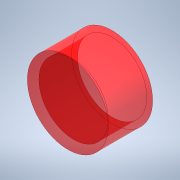
# Autodesk Inventor part: plastic diffuser
Saved by Autodesk Inventor 2022.1 (Build 261234000, 234)
## iProperties
Created: 2019-08-22
Part Number: plastic diffuser
Material: Стекло
Document SubType Name: Modeling
Designer: Иванов Д.А.
Mass: 3.13584 g
Surface Area: 20.169 cm^2
Volume: 1.43846 cm^3
Density: 2.18 g/cm^3
Appearance: Стеклянная лампа — Откл
Author: Иванов Д.А.
Autodesk Inventor part; units mm, degrees
(part 1 of 2)
ref_plane "YZ Plane" through (0, 0, 0) normal (1, 0, 0) x (0, 1, 0)
ref_plane "XZ Plane" through (0, 0, 0) normal (0, 1, 0) x (-1, 0, 0)
ref_plane "XY Plane" through (0, 0, 0) normal (0, 0, 1) x (1, 0, 0)
sketch "Эскиз1" plane through (0, 0, 0) normal (0, 1, 0) x (-1, 0, 0)
  circle A0 centre (0, 0) radius 9
  circle A1 centre (0, 0) radius 10.5
  dimension "d0" = 18
  dimension "d1" = 21
  constraints: 2 centre point, 2 coincident
  measures "d0" diameter of A0
  measures "d1" diameter of A1
extrude "Выдавливание1" add sketch "Эскиз1" along normal blind 10
extrude "Выдавливание2" add sketch "Эскиз1" against normal blind 1.5 contours A0 | A1
sketch "Эскиз3" plane through (0, 10, 0) normal (0, 1, 0) x (1, 0, 0)
  circle A0 centre (0, -9) radius 0.125
  circle A1 centre (0, 0) radius 9 projected
  line L0 (0, -9) -> (0, 0) construction
  line L1 (0, 0) -> (9, 0) construction
  circle A2 centre (0, -8.5) radius 0.125
  circle A3 centre (0, -8) radius 0.125
  circle A4 centre (0, -7.5) radius 0.125
  circle A5 centre (0, -7) radius 0.125
  circle A6 centre (0, -6.5) radius 0.125
  circle A7 centre (0, -6) radius 0.125
  circle A8 centre (0, -5.5) radius 0.125
  circle A9 centre (0, -5) radius 0.125
  circle A10 centre (0, -4.5) radius 0.125
  circle A11 centre (0, -4) radius 0.125
  circle A12 centre (0, -3.5) radius 0.125
  circle A13 centre (0, -3) radius 0.125
  circle A14 centre (0, -2.5) radius 0.125
  circle A15 centre (0, -2) radius 0.125
  circle A16 centre (0, -1.5) radius 0.125
  circle A17 centre (0, -1) radius 0.125
  circle A18 centre (0, -0.5) radius 0.125
  circle A19 centre (0, 0) radius 0.125
  circle A20 centre (0, 0.5) radius 0.125
  circle A21 centre (0, 1) radius 0.125
  circle A22 centre (0, 1.5) radius 0.125
  circle A23 centre (0, 2) radius 0.125
  circle A24 centre (0, 2.5) radius 0.125
  circle A25 centre (0, 3) radius 0.125
  circle A26 centre (0, 3.5) radius 0.125
  circle A27 centre (0, 4) radius 0.125
  circle A28 centre (0, 4.5) radius 0.125
  circle A29 centre (0, 5) radius 0.125
  circle A30 centre (0, 5.5) radius 0.125
  circle A31 centre (0, 6) radius 0.125
  circle A32 centre (0, 6.5) radius 0.125
  circle A33 centre (0, 7) radius 0.125
  circle A34 centre (0, 7.5) radius 0.125
  circle A35 centre (0, 8) radius 0.125
  circle A36 centre (0, 8.5) radius 0.125
  circle A37 centre (0, 9) radius 0.125
  circle A38 centre (0.5, -9) radius 0.125
  circle A39 centre (0.5, -8.5) radius 0.125
  circle A40 centre (0.5, -8) radius 0.125
  circle A41 centre (0.5, -7.5) radius 0.125
  circle A42 centre (0.5, -7) radius 0.125
  circle A43 centre (0.5, -6.5) radius 0.125
  circle A44 centre (0.5, -6) radius 0.125
  circle A45 centre (0.5, -5.5) radius 0.125
  circle A46 centre (0.5, -5) radius 0.125
  circle A47 centre (0.5, -4.5) radius 0.125
  circle A48 centre (0.5, -4) radius 0.125
  circle A49 centre (0.5, -3.5) radius 0.125
  circle A50 centre (0.5, -3) radius 0.125
  circle A51 centre (0.5, -2.5) radius 0.125
  circle A52 centre (0.5, -2) radius 0.125
  circle A53 centre (0.5, -1.5) radius 0.125
  circle A54 centre (0.5, -1) radius 0.125
  circle A55 centre (0.5, -0.5) radius 0.125
  circle A56 centre (0.5, 0) radius 0.125
  circle A57 centre (0.5, 0.5) radius 0.125
  circle A58 centre (0.5, 1) radius 0.125
  circle A59 centre (0.5, 1.5) radius 0.125
  circle A60 centre (0.5, 2) radius 0.125
  circle A61 centre (0.5, 2.5) radius 0.125
  circle A62 centre (0.5, 3) radius 0.125
  circle A63 centre (0.5, 3.5) radius 0.125
  circle A64 centre (0.5, 4) radius 0.125
  circle A65 centre (0.5, 4.5) radius 0.125
  circle A66 centre (0.5, 5) radius 0.125
  circle A67 centre (0.5, 5.5) radius 0.125
  circle A68 centre (0.5, 6) radius 0.125
  circle A69 centre (0.5, 6.5) radius 0.125
  circle A70 centre (0.5, 7) radius 0.125
  circle A71 centre (0.5, 7.5) radius 0.125
  circle A72 centre (0.5, 8) radius 0.125
  circle A73 centre (0.5, 8.5) radius 0.125
  circle A74 centre (0.5, 9) radius 0.125
  circle A75 centre (1, -9) radius 0.125
  circle A76 centre (1, -8.5) radius 0.125
  circle A77 centre (1, -8) radius 0.125
  circle A78 centre (1, -7.5) radius 0.125
  circle A79 centre (1, -7) radius 0.125
  circle A80 centre (1, -6.5) radius 0.125
  circle A81 centre (1, -6) radius 0.125
  circle A82 centre (1, -5.5) radius 0.125
  circle A83 centre (1, -5) radius 0.125
  circle A84 centre (1, -4.5) radius 0.125
  circle A85 centre (1, -4) radius 0.125
  circle A86 centre (1, -3.5) radius 0.125
  circle A87 centre (1, -3) radius 0.125
  circle A88 centre (1, -2.5) radius 0.125
  circle A89 centre (1, -2) radius 0.125
  circle A90 centre (1, -1.5) radius 0.125
  circle A91 centre (1, -1) radius 0.125
  circle A92 centre (1, -0.5) radius 0.125
  circle A93 centre (1, 0) radius 0.125
  circle A94 centre (1, 0.5) radius 0.125
  circle A95 centre (1, 1) radius 0.125
  circle A96 centre (1, 1.5) radius 0.125
  circle A97 centre (1, 2) radius 0.125
  circle A98 centre (1, 2.5) radius 0.125
  circle A99 centre (1, 3) radius 0.125
  circle A100 centre (1, 3.5) radius 0.125
  circle A101 centre (1, 4) radius 0.125
  circle A102 centre (1, 4.5) radius 0.125
  circle A103 centre (1, 5) radius 0.125
  circle A104 centre (1, 5.5) radius 0.125
  circle A105 centre (1, 6) radius 0.125
  circle A106 centre (1, 6.5) radius 0.125
  circle A107 centre (1, 7) radius 0.125
  circle A108 centre (1, 7.5) radius 0.125
  circle A109 centre (1, 8) radius 0.125
  circle A110 centre (1, 8.5) radius 0.125
  circle A111 centre (1, 9) radius 0.125
  circle A112 centre (1.5, -9) radius 0.125
  circle A113 centre (1.5, -8.5) radius 0.125
  circle A114 centre (1.5, -8) radius 0.125
  circle A115 centre (1.5, -7.5) radius 0.125
  circle A116 centre (1.5, -7) radius 0.125
  circle A117 centre (1.5, -6.5) radius 0.125
  circle A118 centre (1.5, -6) radius 0.125
  circle A119 centre (1.5, -5.5) radius 0.125
  circle A120 centre (1.5, -5) radius 0.125
  circle A121 centre (1.5, -4.5) radius 0.125
  circle A122 centre (1.5, -4) radius 0.125
  circle A123 centre (1.5, -3.5) radius 0.125
  circle A124 centre (1.5, -3) radius 0.125
  circle A125 centre (1.5, -2.5) radius 0.125
  circle A126 centre (1.5, -2) radius 0.125
  circle A127 centre (1.5, -1.5) radius 0.125
  circle A128 centre (1.5, -1) radius 0.125
  circle A129 centre (1.5, -0.5) radius 0.125
  circle A130 centre (1.5, 0) radius 0.125
  circle A131 centre (1.5, 0.5) radius 0.125
  circle A132 centre (1.5, 1) radius 0.125
  circle A133 centre (1.5, 1.5) radius 0.125
  circle A134 centre (1.5, 2) radius 0.125
  circle A135 centre (1.5, 2.5) radius 0.125
  circle A136 centre (1.5, 3) radius 0.125
  circle A137 centre (1.5, 3.5) radius 0.125
  circle A138 centre (1.5, 4) radius 0.125
  circle A139 centre (1.5, 4.5) radius 0.125
  circle A140 centre (1.5, 5) radius 0.125
  circle A141 centre (1.5, 5.5) radius 0.125
  circle A142 centre (1.5, 6) radius 0.125
  circle A143 centre (1.5, 6.5) radius 0.125
  circle A144 centre (1.5, 7) radius 0.125
  circle A145 centre (1.5, 7.5) radius 0.125
  circle A146 centre (1.5, 8) radius 0.125
  circle A147 centre (1.5, 8.5) radius 0.125
  circle A148 centre (1.5, 9) radius 0.125
  circle A149 centre (2, -9) radius 0.125
  circle A150 centre (2, -8.5) radius 0.125
  circle A151 centre (2, -8) radius 0.125
  circle A152 centre (2, -7.5) radius 0.125
  circle A153 centre (2, -7) radius 0.125
  circle A154 centre (2, -6.5) radius 0.125
  circle A155 centre (2, -6) radius 0.125
  circle A156 centre (2, -5.5) radius 0.125
  circle A157 centre (2, -5) radius 0.125
  circle A158 centre (2, -4.5) radius 0.125
  circle A159 centre (2, -4) radius 0.125
  circle A160 centre (2, -3.5) radius 0.125
  circle A161 centre (2, -3) radius 0.125
  circle A162 centre (2, -2.5) radius 0.125
  circle A163 centre (2, -2) radius 0.125
  circle A164 centre (2, -1.5) radius 0.125
  circle A165 centre (2, -1) radius 0.125
  circle A166 centre (2, -0.5) radius 0.125
  circle A167 centre (2, 0) radius 0.125
  circle A168 centre (2, 0.5) radius 0.125
  circle A169 centre (2, 1) radius 0.125
  circle A170 centre (2, 1.5) radius 0.125
  circle A171 centre (2, 2) radius 0.125
  circle A172 centre (2, 2.5) radius 0.125
  circle A173 centre (2, 3) radius 0.125
  circle A174 centre (2, 3.5) radius 0.125
  circle A175 centre (2, 4) radius 0.125
  circle A176 centre (2, 4.5) radius 0.125
  circle A177 centre (2, 5) radius 0.125
  circle A178 centre (2, 5.5) radius 0.125
  circle A179 centre (2, 6) radius 0.125
  circle A180 centre (2, 6.5) radius 0.125
  circle A181 centre (2, 7) radius 0.125
  circle A182 centre (2, 7.5) radius 0.125
  circle A183 centre (2, 8) radius 0.125
  circle A184 centre (2, 8.5) radius 0.125
  circle A185 centre (2, 9) radius 0.125
  circle A186 centre (2.5, -9) radius 0.125
  circle A187 centre (2.5, -8.5) radius 0.125
  circle A188 centre (2.5, -8) radius 0.125
  circle A189 centre (2.5, -7.5) radius 0.125
  circle A190 centre (2.5, -7) radius 0.125
  circle A191 centre (2.5, -6.5) radius 0.125
  circle A192 centre (2.5, -6) radius 0.125
  circle A193 centre (2.5, -5.5) radius 0.125
  circle A194 centre (2.5, -5) radius 0.125
  circle A195 centre (2.5, -4.5) radius 0.125
  circle A196 centre (2.5, -4) radius 0.125
  circle A197 centre (2.5, -3.5) radius 0.125
  circle A198 centre (2.5, -3) radius 0.125
  circle A199 centre (2.5, -2.5) radius 0.125
  circle A200 centre (2.5, -2) radius 0.125
  circle A201 centre (2.5, -1.5) radius 0.125
  circle A202 centre (2.5, -1) radius 0.125
  circle A203 centre (2.5, -0.5) radius 0.125
  circle A204 centre (2.5, 0) radius 0.125
  circle A205 centre (2.5, 0.5) radius 0.125
  circle A206 centre (2.5, 1) radius 0.125
  circle A207 centre (2.5, 1.5) radius 0.125
  circle A208 centre (2.5, 2) radius 0.125
  circle A209 centre (2.5, 2.5) radius 0.125
  circle A210 centre (2.5, 3) radius 0.125
  circle A211 centre (2.5, 3.5) radius 0.125
  circle A212 centre (2.5, 4) radius 0.125
  circle A213 centre (2.5, 4.5) radius 0.125
  circle A214 centre (2.5, 5) radius 0.125
  circle A215 centre (2.5, 5.5) radius 0.125
  circle A216 centre (2.5, 6) radius 0.125
  circle A217 centre (2.5, 6.5) radius 0.125
  circle A218 centre (2.5, 7) radius 0.125
  circle A219 centre (2.5, 7.5) radius 0.125
  circle A220 centre (2.5, 8) radius 0.125
  circle A221 centre (2.5, 8.5) radius 0.125
  circle A222 centre (2.5, 9) radius 0.125
  circle A223 centre (3, -9) radius 0.125
  circle A224 centre (3, -8.5) radius 0.125
  circle A225 centre (3, -8) radius 0.125
  circle A226 centre (3, -7.5) radius 0.125
  circle A227 centre (3, -7) radius 0.125
  circle A228 centre (3, -6.5) radius 0.125
  circle A229 centre (3, -6) radius 0.125
  circle A230 centre (3, -5.5) radius 0.125
  circle A231 centre (3, -5) radius 0.125
  circle A232 centre (3, -4.5) radius 0.125
  circle A233 centre (3, -4) radius 0.125
  circle A234 centre (3, -3.5) radius 0.125
  circle A235 centre (3, -3) radius 0.125
  circle A236 centre (3, -2.5) radius 0.125
  circle A237 centre (3, -2) radius 0.125
  circle A238 centre (3, -1.5) radius 0.125
  circle A239 centre (3, -1) radius 0.125
  circle A240 centre (3, -0.5) radius 0.125
  circle A241 centre (3, 0) radius 0.125
  circle A242 centre (3, 0.5) radius 0.125
  circle A243 centre (3, 1) radius 0.125
  circle A244 centre (3, 1.5) radius 0.125
  circle A245 centre (3, 2) radius 0.125
  circle A246 centre (3, 2.5) radius 0.125
  circle A247 centre (3, 3) radius 0.125
  circle A248 centre (3, 3.5) radius 0.125
  circle A249 centre (3, 4) radius 0.125
  circle A250 centre (3, 4.5) radius 0.125
  circle A251 centre (3, 5) radius 0.125
  circle A252 centre (3, 5.5) radius 0.125
  circle A253 centre (3, 6) radius 0.125
  circle A254 centre (3, 6.5) radius 0.125
  circle A255 centre (3, 7) radius 0.125
  circle A256 centre (3, 7.5) radius 0.125
  circle A257 centre (3, 8) radius 0.125
  circle A258 centre (3, 8.5) radius 0.125
  circle A259 centre (3, 9) radius 0.125
  circle A260 centre (3.5, -9) radius 0.125
  circle A261 centre (3.5, -8.5) radius 0.125
  circle A262 centre (3.5, -8) radius 0.125
  circle A263 centre (3.5, -7.5) radius 0.125
  circle A264 centre (3.5, -7) radius 0.125
  circle A265 centre (3.5, -6.5) radius 0.125
  circle A266 centre (3.5, -6) radius 0.125
  circle A267 centre (3.5, -5.5) radius 0.125
  circle A268 centre (3.5, -5) radius 0.125
  circle A269 centre (3.5, -4.5) radius 0.125
  circle A270 centre (3.5, -4) radius 0.125
  circle A271 centre (3.5, -3.5) radius 0.125
  circle A272 centre (3.5, -3) radius 0.125
  circle A273 centre (3.5, -2.5) radius 0.125
  circle A274 centre (3.5, -2) radius 0.125
  circle A275 centre (3.5, -1.5) radius 0.125
  circle A276 centre (3.5, -1) radius 0.125
  circle A277 centre (3.5, -0.5) radius 0.125
  circle A278 centre (3.5, 0) radius 0.125
  circle A279 centre (3.5, 0.5) radius 0.125
  circle A280 centre (3.5, 1) radius 0.125
  circle A281 centre (3.5, 1.5) radius 0.125
  circle A282 centre (3.5, 2) radius 0.125
  circle A283 centre (3.5, 2.5) radius 0.125
  circle A284 centre (3.5, 3) radius 0.125
  circle A285 centre (3.5, 3.5) radius 0.125
  circle A286 centre (3.5, 4) radius 0.125
  circle A287 centre (3.5, 4.5) radius 0.125
  circle A288 centre (3.5, 5) radius 0.125
  circle A289 centre (3.5, 5.5) radius 0.125
  circle A290 centre (3.5, 6) radius 0.125
  circle A291 centre (3.5, 6.5) radius 0.125
  circle A292 centre (3.5, 7) radius 0.125
  circle A293 centre (3.5, 7.5) radius 0.125
  circle A294 centre (3.5, 8) radius 0.125
  circle A295 centre (3.5, 8.5) radius 0.125
  circle A296 centre (3.5, 9) radius 0.125
  circle A297 centre (4, -9) radius 0.125
  circle A298 centre (4, -8.5) radius 0.125
  circle A299 centre (4, -8) radius 0.125
  circle A300 centre (4, -7.5) radius 0.125
  circle A301 centre (4, -7) radius 0.125
  circle A302 centre (4, -6.5) radius 0.125
  circle A303 centre (4, -6) radius 0.125
  circle A304 centre (4, -5.5) radius 0.125
  circle A305 centre (4, -5) radius 0.125
  circle A306 centre (4, -4.5) radius 0.125
  circle A307 centre (4, -4) radius 0.125
  circle A308 centre (4, -3.5) radius 0.125
  circle A309 centre (4, -3) radius 0.125
  circle A310 centre (4, -2.5) radius 0.125
  circle A311 centre (4, -2) radius 0.125
  circle A312 centre (4, -1.5) radius 0.125
  circle A313 centre (4, -1) radius 0.125
  circle A314 centre (4, -0.5) radius 0.125
  circle A315 centre (4, 0) radius 0.125
  circle A316 centre (4, 0.5) radius 0.125
  circle A317 centre (4, 1) radius 0.125
  circle A318 centre (4, 1.5) radius 0.125
  circle A319 centre (4, 2) radius 0.125
  circle A320 centre (4, 2.5) radius 0.125
  circle A321 centre (4, 3) radius 0.125
  circle A322 centre (4, 3.5) radius 0.125
  circle A323 centre (4, 4) radius 0.125
  circle A324 centre (4, 4.5) radius 0.125
  circle A325 centre (4, 5) radius 0.125
  circle A326 centre (4, 5.5) radius 0.125
  circle A327 centre (4, 6) radius 0.125
  circle A328 centre (4, 6.5) radius 0.125
  circle A329 centre (4, 7) radius 0.125
  circle A330 centre (4, 7.5) radius 0.125
  circle A331 centre (4, 8) radius 0.125
  circle A332 centre (4, 8.5) radius 0.125
  circle A333 centre (4, 9) radius 0.125
  circle A334 centre (4.5, -9) radius 0.125
  circle A335 centre (4.5, -8.5) radius 0.125
  circle A336 centre (4.5, -8) radius 0.125
  circle A337 centre (4.5, -7.5) radius 0.125
  circle A338 centre (4.5, -7) radius 0.125
  circle A339 centre (4.5, -6.5) radius 0.125
  circle A340 centre (4.5, -6) radius 0.125
  circle A341 centre (4.5, -5.5) radius 0.125
  circle A342 centre (4.5, -5) radius 0.125
  circle A343 centre (4.5, -4.5) radius 0.125
  circle A344 centre (4.5, -4) radius 0.125
  circle A345 centre (4.5, -3.5) radius 0.125
  circle A346 centre (4.5, -3) radius 0.125
  circle A347 centre (4.5, -2.5) radius 0.125
  circle A348 centre (4.5, -2) radius 0.125
  circle A349 centre (4.5, -1.5) radius 0.125
  circle A350 centre (4.5, -1) radius 0.125
  circle A351 centre (4.5, -0.5) radius 0.125
  circle A352 centre (4.5, 0) radius 0.125
  circle A353 centre (4.5, 0.5) radius 0.125
  circle A354 centre (4.5, 1) radius 0.125
  circle A355 centre (4.5, 1.5) radius 0.125
  circle A356 centre (4.5, 2) radius 0.125
  circle A357 centre (4.5, 2.5) radius 0.125
  circle A358 centre (4.5, 3) radius 0.125
  circle A359 centre (4.5, 3.5) radius 0.125
  circle A360 centre (4.5, 4) radius 0.125
  circle A361 centre (4.5, 4.5) radius 0.125
  circle A362 centre (4.5, 5) radius 0.125
  circle A363 centre (4.5, 5.5) radius 0.125
  circle A364 centre (4.5, 6) radius 0.125
  circle A365 centre (4.5, 6.5) radius 0.125
  circle A366 centre (4.5, 7) radius 0.125
  circle A367 centre (4.5, 7.5) radius 0.125
  circle A368 centre (4.5, 8) radius 0.125
  circle A369 centre (4.5, 8.5) radius 0.125
  circle A370 centre (4.5, 9) radius 0.125
  circle A371 centre (5, -9) radius 0.125
  circle A372 centre (5, -8.5) radius 0.125
  circle A373 centre (5, -8) radius 0.125
  circle A374 centre (5, -7.5) radius 0.125
  circle A375 centre (5, -7) radius 0.125
  circle A376 centre (5, -6.5) radius 0.125
  circle A377 centre (5, -6) radius 0.125
  circle A378 centre (5, -5.5) radius 0.125
  circle A379 centre (5, -5) radius 0.125
  circle A380 centre (5, -4.5) radius 0.125
  circle A381 centre (5, -4) radius 0.125
  circle A382 centre (5, -3.5) radius 0.125
  circle A383 centre (5, -3) radius 0.125
  circle A384 centre (5, -2.5) radius 0.125
  circle A385 centre (5, -2) radius 0.125
  circle A386 centre (5, -1.5) radius 0.125
  circle A387 centre (5, -1) radius 0.125
  circle A388 centre (5, -0.5) radius 0.125
  circle A389 centre (5, 0) radius 0.125
  circle A390 centre (5, 0.5) radius 0.125
  circle A391 centre (5, 1) radius 0.125
  circle A392 centre (5, 1.5) radius 0.125
  circle A393 centre (5, 2) radius 0.125
  circle A394 centre (5, 2.5) radius 0.125
  circle A395 centre (5, 3) radius 0.125
  circle A396 centre (5, 3.5) radius 0.125
  circle A397 centre (5, 4) radius 0.125
  circle A398 centre (5, 4.5) radius 0.125
  circle A399 centre (5, 5) radius 0.125
  circle A400 centre (5, 5.5) radius 0.125
  circle A401 centre (5, 6) radius 0.125
  circle A402 centre (5, 6.5) radius 0.125
  circle A403 centre (5, 7) radius 0.125
  circle A404 centre (5, 7.5) radius 0.125
  circle A405 centre (5, 8) radius 0.125
  circle A406 centre (5, 8.5) radius 0.125
  circle A407 centre (5, 9) radius 0.125
  circle A408 centre (5.5, -9) radius 0.125
  circle A409 centre (5.5, -8.5) radius 0.125
  circle A410 centre (5.5, -8) radius 0.125
  circle A411 centre (5.5, -7.5) radius 0.125
  circle A412 centre (5.5, -7) radius 0.125
  circle A413 centre (5.5, -6.5) radius 0.125
  circle A414 centre (5.5, -6) radius 0.125
  circle A415 centre (5.5, -5.5) radius 0.125
  circle A416 centre (5.5, -5) radius 0.125
  circle A417 centre (5.5, -4.5) radius 0.125
  circle A418 centre (5.5, -4) radius 0.125
  circle A419 centre (5.5, -3.5) radius 0.125
  circle A420 centre (5.5, -3) radius 0.125
  circle A421 centre (5.5, -2.5) radius 0.125
  circle A422 centre (5.5, -2) radius 0.125
  circle A423 centre (5.5, -1.5) radius 0.125
  circle A424 centre (5.5, -1) radius 0.125
  circle A425 centre (5.5, -0.5) radius 0.125
  circle A426 centre (5.5, 0) radius 0.125
  circle A427 centre (5.5, 0.5) radius 0.125
  circle A428 centre (5.5, 1) radius 0.125
  circle A429 centre (5.5, 1.5) radius 0.125
  circle A430 centre (5.5, 2) radius 0.125
  circle A431 centre (5.5, 2.5) radius 0.125
  circle A432 centre (5.5, 3) radius 0.125
  circle A433 centre (5.5, 3.5) radius 0.125
  circle A434 centre (5.5, 4) radius 0.125
  circle A435 centre (5.5, 4.5) radius 0.125
  circle A436 centre (5.5, 5) radius 0.125
  circle A437 centre (5.5, 5.5) radius 0.125
  circle A438 centre (5.5, 6) radius 0.125
  circle A439 centre (5.5, 6.5) radius 0.125
  circle A440 centre (5.5, 7) radius 0.125
  circle A441 centre (5.5, 7.5) radius 0.125
  circle A442 centre (5.5, 8) radius 0.125
  circle A443 centre (5.5, 8.5) radius 0.125
  circle A444 centre (5.5, 9) radius 0.125
  circle A445 centre (6, -9) radius 0.125
  circle A446 centre (6, -8.5) radius 0.125
  circle A447 centre (6, -8) radius 0.125
  circle A448 centre (6, -7.5) radius 0.125
  circle A449 centre (6, -7) radius 0.125
  circle A450 centre (6, -6.5) radius 0.125
  circle A451 centre (6, -6) radius 0.125
  circle A452 centre (6, -5.5) radius 0.125
  circle A453 centre (6, -5) radius 0.125
  circle A454 centre (6, -4.5) radius 0.125
  circle A455 centre (6, -4) radius 0.125
  circle A456 centre (6, -3.5) radius 0.125
  circle A457 centre (6, -3) radius 0.125
  circle A458 centre (6, -2.5) radius 0.125
  circle A459 centre (6, -2) radius 0.125
  circle A460 centre (6, -1.5) radius 0.125
  circle A461 centre (6, -1) radius 0.125
  circle A462 centre (6, -0.5) radius 0.125
  circle A463 centre (6, 0) radius 0.125
  circle A464 centre (6, 0.5) radius 0.125
  circle A465 centre (6, 1) radius 0.125
  circle A466 centre (6, 1.5) radius 0.125
  circle A467 centre (6, 2) radius 0.125
  circle A468 centre (6, 2.5) radius 0.125
  circle A469 centre (6, 3) radius 0.125
  circle A470 centre (6, 3.5) radius 0.125
  circle A471 centre (6, 4) radius 0.125
  circle A472 centre (6, 4.5) radius 0.125
  circle A473 centre (6, 5) radius 0.125
  circle A474 centre (6, 5.5) radius 0.125
  circle A475 centre (6, 6) radius 0.125
  circle A476 centre (6, 6.5) radius 0.125
  circle A477 centre (6, 7) radius 0.125
  circle A478 centre (6, 7.5) radius 0.125
  circle A479 centre (6, 8) radius 0.125
  circle A480 centre (6, 8.5) radius 0.125
  circle A481 centre (6, 9) radius 0.125
  circle A482 centre (6.5, -9) radius 0.125
  circle A483 centre (6.5, -8.5) radius 0.125
  circle A484 centre (6.5, -8) radius 0.125
  circle A485 centre (6.5, -7.5) radius 0.125
  circle A486 centre (6.5, -7) radius 0.125
  circle A487 centre (6.5, -6.5) radius 0.125
  circle A488 centre (6.5, -6) radius 0.125
  circle A489 centre (6.5, -5.5) radius 0.125
  circle A490 centre (6.5, -5) radius 0.125
  circle A491 centre (6.5, -4.5) radius 0.125
  circle A492 centre (6.5, -4) radius 0.125
  circle A493 centre (6.5, -3.5) radius 0.125
  circle A494 centre (6.5, -3) radius 0.125
  circle A495 centre (6.5, -2.5) radius 0.125
  circle A496 centre (6.5, -2) radius 0.125
  circle A497 centre (6.5, -1.5) radius 0.125
  circle A498 centre (6.5, -1) radius 0.125
  circle A499 centre (6.5, -0.5) radius 0.125
  circle A500 centre (6.5, 0) radius 0.125
  circle A501 centre (6.5, 0.5) radius 0.125
  circle A502 centre (6.5, 1) radius 0.125
  circle A503 centre (6.5, 1.5) radius 0.125
  circle A504 centre (6.5, 2) radius 0.125
  circle A505 centre (6.5, 2.5) radius 0.125
  circle A506 centre (6.5, 3) radius 0.125
  circle A507 centre (6.5, 3.5) radius 0.125
  circle A508 centre (6.5, 4) radius 0.125
  circle A509 centre (6.5, 4.5) radius 0.125
  circle A510 centre (6.5, 5) radius 0.125
  circle A511 centre (6.5, 5.5) radius 0.125
  circle A512 centre (6.5, 6) radius 0.125
  circle A513 centre (6.5, 6.5) radius 0.125
  circle A514 centre (6.5, 7) radius 0.125
  circle A515 centre (6.5, 7.5) radius 0.125
  circle A516 centre (6.5, 8) radius 0.125
  circle A517 centre (6.5, 8.5) radius 0.125
  circle A518 centre (6.5, 9) radius 0.125
  circle A519 centre (7, -9) radius 0.125
  circle A520 centre (7, -8.5) radius 0.125
  circle A521 centre (7, -8) radius 0.125
  circle A522 centre (7, -7.5) radius 0.125
  circle A523 centre (7, -7) radius 0.125
  circle A524 centre (7, -6.5) radius 0.125
  circle A525 centre (7, -6) radius 0.125
  circle A526 centre (7, -5.5) radius 0.125
  circle A527 centre (7, -5) radius 0.125
  circle A528 centre (7, -4.5) radius 0.125
  circle A529 centre (7, -4) radius 0.125
  circle A530 centre (7, -3.5) radius 0.125
  circle A531 centre (7, -3) radius 0.125
  circle A532 centre (7, -2.5) radius 0.125
  circle A533 centre (7, -2) radius 0.125
  circle A534 centre (7, -1.5) radius 0.125
  circle A535 centre (7, -1) radius 0.125
  circle A536 centre (7, -0.5) radius 0.125
  circle A537 centre (7, 0) radius 0.125
  circle A538 centre (7, 0.5) radius 0.125
  circle A539 centre (7, 1) radius 0.125
  circle A540 centre (7, 1.5) radius 0.125
  circle A541 centre (7, 2) radius 0.125
  circle A542 centre (7, 2.5) radius 0.125
  circle A543 centre (7, 3) radius 0.125
  circle A544 centre (7, 3.5) radius 0.125
  circle A545 centre (7, 4) radius 0.125
  circle A546 centre (7, 4.5) radius 0.125
  circle A547 centre (7, 5) radius 0.125
  circle A548 centre (7, 5.5) radius 0.125
  circle A549 centre (7, 6) radius 0.125
  circle A550 centre (7, 6.5) radius 0.125
  circle A551 centre (7, 7) radius 0.125
  circle A552 centre (7, 7.5) radius 0.125
  circle A553 centre (7, 8) radius 0.125
  circle A554 centre (7, 8.5) radius 0.125
  circle A555 centre (7, 9) radius 0.125
  circle A556 centre (7.5, -9) radius 0.125
  circle A557 centre (7.5, -8.5) radius 0.125
  circle A558 centre (7.5, -8) radius 0.125
  circle A559 centre (7.5, -7.5) radius 0.125
  circle A560 centre (7.5, -7) radius 0.125
  circle A561 centre (7.5, -6.5) radius 0.125
  circle A562 centre (7.5, -6) radius 0.125
  circle A563 centre (7.5, -5.5) radius 0.125
  circle A564 centre (7.5, -5) radius 0.125
  circle A565 centre (7.5, -4.5) radius 0.125
  circle A566 centre (7.5, -4) radius 0.125
  circle A567 centre (7.5, -3.5) radius 0.125
  circle A568 centre (7.5, -3) radius 0.125
  circle A569 centre (7.5, -2.5) radius 0.125
  circle A570 centre (7.5, -2) radius 0.125
  circle A571 centre (7.5, -1.5) radius 0.125
  circle A572 centre (7.5, -1) radius 0.125
  circle A573 centre (7.5, -0.5) radius 0.125
  circle A574 centre (7.5, 0) radius 0.125
  circle A575 centre (7.5, 0.5) radius 0.125
  circle A576 centre (7.5, 1) radius 0.125
  circle A577 centre (7.5, 1.5) radius 0.125
  circle A578 centre (7.5, 2) radius 0.125
  circle A579 centre (7.5, 2.5) radius 0.125
  circle A580 centre (7.5, 3) radius 0.125
  circle A581 centre (7.5, 3.5) radius 0.125
  circle A582 centre (7.5, 4) radius 0.125
  circle A583 centre (7.5, 4.5) radius 0.125
  circle A584 centre (7.5, 5) radius 0.125
  circle A585 centre (7.5, 5.5) radius 0.125
  circle A586 centre (7.5, 6) radius 0.125
  circle A587 centre (7.5, 6.5) radius 0.125
  circle A588 centre (7.5, 7) radius 0.125
  circle A589 centre (7.5, 7.5) radius 0.125
  circle A590 centre (7.5, 8) radius 0.125
  circle A591 centre (7.5, 8.5) radius 0.125
  circle A592 centre (7.5, 9) radius 0.125
  circle A593 centre (8, -9) radius 0.125
  circle A594 centre (8, -8.5) radius 0.125
  circle A595 centre (8, -8) radius 0.125
  circle A596 centre (8, -7.5) radius 0.125
  circle A597 centre (8, -7) radius 0.125
  circle A598 centre (8, -6.5) radius 0.125
  circle A599 centre (8, -6) radius 0.125
  circle A600 centre (8, -5.5) radius 0.125
  circle A601 centre (8, -5) radius 0.125
  circle A602 centre (8, -4.5) radius 0.125
  circle A603 centre (8, -4) radius 0.125
  circle A604 centre (8, -3.5) radius 0.125
  circle A605 centre (8, -3) radius 0.125
  circle A606 centre (8, -2.5) radius 0.125
  circle A607 centre (8, -2) radius 0.125
  circle A608 centre (8, -1.5) radius 0.125
  circle A609 centre (8, -1) radius 0.125
  circle A610 centre (8, -0.5) radius 0.125
  circle A611 centre (8, 0) radius 0.125
  circle A612 centre (8, 0.5) radius 0.125
  circle A613 centre (8, 1) radius 0.125
  circle A614 centre (8, 1.5) radius 0.125
  circle A615 centre (8, 2) radius 0.125
  circle A616 centre (8, 2.5) radius 0.125
  circle A617 centre (8, 3) radius 0.125
  circle A618 centre (8, 3.5) radius 0.125
  circle A619 centre (8, 4) radius 0.125
  circle A620 centre (8, 4.5) radius 0.125
  circle A621 centre (8, 5) radius 0.125
  circle A622 centre (8, 5.5) radius 0.125
  circle A623 centre (8, 6) radius 0.125
  circle A624 centre (8, 6.5) radius 0.125
  circle A625 centre (8, 7) radius 0.125
  circle A626 centre (8, 7.5) radius 0.125
  circle A627 centre (8, 8) radius 0.125
  circle A628 centre (8, 8.5) radius 0.125
  circle A629 centre (8, 9) radius 0.125
  circle A630 centre (8.5, -9) radius 0.125
  circle A631 centre (8.5, -8.5) radius 0.125
  circle A632 centre (8.5, -8) radius 0.125
  circle A633 centre (8.5, -7.5) radius 0.125
  circle A634 centre (8.5, -7) radius 0.125
  circle A635 centre (8.5, -6.5) radius 0.125
  circle A636 centre (8.5, -6) radius 0.125
  circle A637 centre (8.5, -5.5) radius 0.125
  circle A638 centre (8.5, -5) radius 0.125
  circle A639 centre (8.5, -4.5) radius 0.125
  circle A640 centre (8.5, -4) radius 0.125
  circle A641 centre (8.5, -3.5) radius 0.125
  circle A642 centre (8.5, -3) radius 0.125
  circle A643 centre (8.5, -2.5) radius 0.125
  circle A644 centre (8.5, -2) radius 0.125
  circle A645 centre (8.5, -1.5) radius 0.125
  circle A646 centre (8.5, -1) radius 0.125
  circle A647 centre (8.5, -0.5) radius 0.125
  circle A648 centre (8.5, 0) radius 0.125
  circle A649 centre (8.5, 0.5) radius 0.125
  circle A650 centre (8.5, 1) radius 0.125
  circle A651 centre (8.5, 1.5) radius 0.125
  circle A652 centre (8.5, 2) radius 0.125
  circle A653 centre (8.5, 2.5) radius 0.125
  circle A654 centre (8.5, 3) radius 0.125
  circle A655 centre (8.5, 3.5) radius 0.125
  circle A656 centre (8.5, 4) radius 0.125
  circle A657 centre (8.5, 4.5) radius 0.125
  circle A658 centre (8.5, 5) radius 0.125
  circle A659 centre (8.5, 5.5) radius 0.125
  circle A660 centre (8.5, 6) radius 0.125
  circle A661 centre (8.5, 6.5) radius 0.125
  circle A662 centre (8.5, 7) radius 0.125
  circle A663 centre (8.5, 7.5) radius 0.125
  circle A664 centre (8.5, 8) radius 0.125
  circle A665 centre (8.5, 8.5) radius 0.125
  circle A666 centre (8.5, 9) radius 0.125
  circle A667 centre (9, -9) radius 0.125
  circle A668 centre (9, -8.5) radius 0.125
  circle A669 centre (9, -8) radius 0.125
  circle A670 centre (9, -7.5) radius 0.125
  circle A671 centre (9, -7) radius 0.125
  circle A672 centre (9, -6.5) radius 0.125
  circle A673 centre (9, -6) radius 0.125
  circle A674 centre (9, -5.5) radius 0.125
  circle A675 centre (9, -5) radius 0.125
  circle A676 centre (9, -4.5) radius 0.125
  circle A677 centre (9, -4) radius 0.125
  circle A678 centre (9, -3.5) radius 0.125
  circle A679 centre (9, -3) radius 0.125
  circle A680 centre (9, -2.5) radius 0.125
  circle A681 centre (9, -2) radius 0.125
  circle A682 centre (9, -1.5) radius 0.125
  circle A683 centre (9, -1) radius 0.125
  circle A684 centre (9, -0.5) radius 0.125
  circle A685 centre (9, 0) radius 0.125
  circle A686 centre (9, 0.5) radius 0.125
  circle A687 centre (9, 1) radius 0.125
  circle A688 centre (9, 1.5) radius 0.125
  circle A689 centre (9, 2) radius 0.125
  circle A690 centre (9, 2.5) radius 0.125
  circle A691 centre (9, 3) radius 0.125
  circle A692 centre (9, 3.5) radius 0.125
  circle A693 centre (9, 4) radius 0.125
  circle A694 centre (9, 4.5) radius 0.125
  circle A695 centre (9, 5) radius 0.125
  circle A696 centre (9, 5.5) radius 0.125
  circle A697 centre (9, 6) radius 0.125
  circle A698 centre (9, 6.5) radius 0.125
  circle A699 centre (9, 7) radius 0.125
  circle A700 centre (9, 7.5) radius 0.125
  circle A701 centre (9, 8) radius 0.125
  circle A702 centre (9, 8.5) radius 0.125
  circle A703 centre (9, 9) radius 0.125
  line L2 (-0.5, -9) -> (-0.5, 0) construction
  circle A704 centre (-0.5, -5.5) radius 0.125
  circle A705 centre (-0.5, -5) radius 0.125
  circle A706 centre (-0.5, -3.5) radius 0.125
  circle A707 centre (-0.5, -4) radius 0.125
  circle A708 centre (-0.5, -4.5) radius 0.125
  circle A709 centre (-0.5, -7.5) radius 0.125
  circle A710 centre (-0.5, -7) radius 0.125
  circle A711 centre (-0.5, -6.5) radius 0.125
  circle A712 centre (-0.5, -6) radius 0.125
  circle A713 centre (-0.5, -3) radius 0.125
  circle A714 centre (-0.5, -2.5) radius 0.125
  circle A715 centre (-0.5, -2) radius 0.125
  circle A716 centre (-0.5, -1.5) radius 0.125
  circle A717 centre (-0.5, 0) radius 0.125
  circle A718 centre (-0.5, -0.5) radius 0.125
  circle A719 centre (-0.5, -1) radius 0.125
  circle A720 centre (-0.5, -9) radius 0.125
  circle A721 centre (-0.5, -8.5) radius 0.125
  circle A722 centre (-0.5, -8) radius 0.125
  circle A723 centre (-0.5, 3.5) radius 0.125
  circle A724 centre (-0.5, 4) radius 0.125
  circle A725 centre (-0.5, 4.5) radius 0.125
  circle A726 centre (-0.5, 7) radius 0.125
  circle A727 centre (-0.5, 7.5) radius 0.125
  circle A728 centre (-0.5, 8) radius 0.125
  circle A729 centre (-0.5, 8.5) radius 0.125
  circle A730 centre (-0.5, 9) radius 0.125
  circle A731 centre (-0.5, 0.5) radius 0.125
  circle A732 centre (-0.5, 1) radius 0.125
  circle A733 centre (-0.5, 1.5) radius 0.125
  circle A734 centre (-0.5, 2) radius 0.125
  circle A735 centre (-0.5, 2.5) radius 0.125
  circle A736 centre (-0.5, 3) radius 0.125
  circle A737 centre (-0.5, 5) radius 0.125
  circle A738 centre (-0.5, 5.5) radius 0.125
  circle A739 centre (-0.5, 6) radius 0.125
  circle A740 centre (-0.5, 6.5) radius 0.125
  line L3 (-1, -9) -> (-1, 0) construction
  circle A741 centre (-1, -5.5) radius 0.125
  circle A742 centre (-1, -5) radius 0.125
  circle A743 centre (-1, -3.5) radius 0.125
  circle A744 centre (-1, -4) radius 0.125
  circle A745 centre (-1, -4.5) radius 0.125
  circle A746 centre (-1, -7.5) radius 0.125
  circle A747 centre (-1, -7) radius 0.125
  circle A748 centre (-1, -6.5) radius 0.125
  circle A749 centre (-1, -6) radius 0.125
  circle A750 centre (-1, -3) radius 0.125
  circle A751 centre (-1, -2.5) radius 0.125
  circle A752 centre (-1, -2) radius 0.125
  circle A753 centre (-1, -1.5) radius 0.125
  circle A754 centre (-1, 0) radius 0.125
  circle A755 centre (-1, -0.5) radius 0.125
  circle A756 centre (-1, -1) radius 0.125
  circle A757 centre (-1, -9) radius 0.125
  circle A758 centre (-1, -8.5) radius 0.125
  circle A759 centre (-1, -8) radius 0.125
  circle A760 centre (-1, 3.5) radius 0.125
  circle A761 centre (-1, 4) radius 0.125
  circle A762 centre (-1, 4.5) radius 0.125
  circle A763 centre (-1, 7) radius 0.125
  circle A764 centre (-1, 7.5) radius 0.125
  circle A765 centre (-1, 8) radius 0.125
  circle A766 centre (-1, 8.5) radius 0.125
  circle A767 centre (-1, 9) radius 0.125
  circle A768 centre (-1, 0.5) radius 0.125
  circle A769 centre (-1, 1) radius 0.125
  circle A770 centre (-1, 1.5) radius 0.125
  circle A771 centre (-1, 2) radius 0.125
  circle A772 centre (-1, 2.5) radius 0.125
  circle A773 centre (-1, 3) radius 0.125
  circle A774 centre (-1, 5) radius 0.125
  circle A775 centre (-1, 5.5) radius 0.125
  circle A776 centre (-1, 6) radius 0.125
  circle A777 centre (-1, 6.5) radius 0.125
  line L4 (-1.5, -9) -> (-1.5, 0) construction
  circle A778 centre (-1.5, -5.5) radius 0.125
  circle A779 centre (-1.5, -5) radius 0.125
  circle A780 centre (-1.5, -3.5) radius 0.125
  circle A781 centre (-1.5, -4) radius 0.125
  circle A782 centre (-1.5, -4.5) radius 0.125
  circle A783 centre (-1.5, -7.5) radius 0.125
  circle A784 centre (-1.5, -7) radius 0.125
  circle A785 centre (-1.5, -6.5) radius 0.125
  circle A786 centre (-1.5, -6) radius 0.125
  circle A787 centre (-1.5, -3) radius 0.125
  circle A788 centre (-1.5, -2.5) radius 0.125
  circle A789 centre (-1.5, -2) radius 0.125
  circle A790 centre (-1.5, -1.5) radius 0.125
  circle A791 centre (-1.5, 0) radius 0.125
  circle A792 centre (-1.5, -0.5) radius 0.125
  circle A793 centre (-1.5, -1) radius 0.125
  circle A794 centre (-1.5, -9) radius 0.125
  circle A795 centre (-1.5, -8.5) radius 0.125
  circle A796 centre (-1.5, -8) radius 0.125
  circle A797 centre (-1.5, 3.5) radius 0.125
  circle A798 centre (-1.5, 4) radius 0.125
  circle A799 centre (-1.5, 4.5) radius 0.125
  circle A800 centre (-1.5, 7) radius 0.125
  circle A801 centre (-1.5, 7.5) radius 0.125
  circle A802 centre (-1.5, 8) radius 0.125
  circle A803 centre (-1.5, 8.5) radius 0.125
  circle A804 centre (-1.5, 9) radius 0.125
  circle A805 centre (-1.5, 0.5) radius 0.125
  circle A806 centre (-1.5, 1) radius 0.125
  circle A807 centre (-1.5, 1.5) radius 0.125
  circle A808 centre (-1.5, 2) radius 0.125
  circle A809 centre (-1.5, 2.5) radius 0.125
  circle A810 centre (-1.5, 3) radius 0.125
  circle A811 centre (-1.5, 5) radius 0.125
  circle A812 centre (-1.5, 5.5) radius 0.125
  circle A813 centre (-1.5, 6) radius 0.125
  circle A814 centre (-1.5, 6.5) radius 0.125
  line L5 (-2, -9) -> (-2, 0) construction
  circle A815 centre (-2, -5.5) radius 0.125
  circle A816 centre (-2, -5) radius 0.125
  circle A817 centre (-2, -3.5) radius 0.125
  circle A818 centre (-2, -4) radius 0.125
  circle A819 centre (-2, -4.5) radius 0.125
  circle A820 centre (-2, -7.5) radius 0.125
  circle A821 centre (-2, -7) radius 0.125
  circle A822 centre (-2, -6.5) radius 0.125
  circle A823 centre (-2, -6) radius 0.125
  circle A824 centre (-2, -3) radius 0.125
  circle A825 centre (-2, -2.5) radius 0.125
  circle A826 centre (-2, -2) radius 0.125
  circle A827 centre (-2, -1.5) radius 0.125
  circle A828 centre (-2, 0) radius 0.125
  circle A829 centre (-2, -0.5) radius 0.125
  circle A830 centre (-2, -1) radius 0.125
  circle A831 centre (-2, -9) radius 0.125
  circle A832 centre (-2, -8.5) radius 0.125
  circle A833 centre (-2, -8) radius 0.125
  circle A834 centre (-2, 3.5) radius 0.125
  circle A835 centre (-2, 4) radius 0.125
  circle A836 centre (-2, 4.5) radius 0.125
  circle A837 centre (-2, 7) radius 0.125
  circle A838 centre (-2, 7.5) radius 0.125
  circle A839 centre (-2, 8) radius 0.125
  circle A840 centre (-2, 8.5) radius 0.125
  circle A841 centre (-2, 9) radius 0.125
  circle A842 centre (-2, 0.5) radius 0.125
  circle A843 centre (-2, 1) radius 0.125
  circle A844 centre (-2, 1.5) radius 0.125
  circle A845 centre (-2, 2) radius 0.125
  circle A846 centre (-2, 2.5) radius 0.125
  circle A847 centre (-2, 3) radius 0.125
  circle A848 centre (-2, 5) radius 0.125
  circle A849 centre (-2, 5.5) radius 0.125
  circle A850 centre (-2, 6) radius 0.125
  circle A851 centre (-2, 6.5) radius 0.125
  line L6 (-2.5, -9) -> (-2.5, 0) construction
  circle A852 centre (-2.5, -5.5) radius 0.125
  circle A853 centre (-2.5, -5) radius 0.125
  circle A854 centre (-2.5, -3.5) radius 0.125
  circle A855 centre (-2.5, -4) radius 0.125
  circle A856 centre (-2.5, -4.5) radius 0.125
  circle A857 centre (-2.5, -7.5) radius 0.125
  circle A858 centre (-2.5, -7) radius 0.125
  circle A859 centre (-2.5, -6.5) radius 0.125
  circle A860 centre (-2.5, -6) radius 0.125
  circle A861 centre (-2.5, -3) radius 0.125
  circle A862 centre (-2.5, -2.5) radius 0.125
  circle A863 centre (-2.5, -2) radius 0.125
  circle A864 centre (-2.5, -1.5) radius 0.125
  circle A865 centre (-2.5, 0) radius 0.125
  circle A866 centre (-2.5, -0.5) radius 0.125
  circle A867 centre (-2.5, -1) radius 0.125
  circle A868 centre (-2.5, -9) radius 0.125
  circle A869 centre (-2.5, -8.5) radius 0.125
  circle A870 centre (-2.5, -8) radius 0.125
  circle A871 centre (-2.5, 3.5) radius 0.125
  circle A872 centre (-2.5, 4) radius 0.125
  circle A873 centre (-2.5, 4.5) radius 0.125
  circle A874 centre (-2.5, 7) radius 0.125
  circle A875 centre (-2.5, 7.5) radius 0.125
  circle A876 centre (-2.5, 8) radius 0.125
  circle A877 centre (-2.5, 8.5) radius 0.125
  circle A878 centre (-2.5, 9) radius 0.125
  circle A879 centre (-2.5, 0.5) radius 0.125
  circle A880 centre (-2.5, 1) radius 0.125
  circle A881 centre (-2.5, 1.5) radius 0.125
  circle A882 centre (-2.5, 2) radius 0.125
  circle A883 centre (-2.5, 2.5) radius 0.125
  circle A884 centre (-2.5, 3) radius 0.125
  circle A885 centre (-2.5, 5) radius 0.125
  circle A886 centre (-2.5, 5.5) radius 0.125
  circle A887 centre (-2.5, 6) radius 0.125
  circle A888 centre (-2.5, 6.5) radius 0.125
  line L7 (-3, -9) -> (-3, 0) construction
  circle A889 centre (-3, -5.5) radius 0.125
  circle A890 centre (-3, -5) radius 0.125
  circle A891 centre (-3, -3.5) radius 0.125
  circle A892 centre (-3, -4) radius 0.125
  circle A893 centre (-3, -4.5) radius 0.125
  circle A894 centre (-3, -7.5) radius 0.125
  circle A895 centre (-3, -7) radius 0.125
  circle A896 centre (-3, -6.5) radius 0.125
  circle A897 centre (-3, -6) radius 0.125
  circle A898 centre (-3, -3) radius 0.125
  circle A899 centre (-3, -2.5) radius 0.125
  circle A900 centre (-3, -2) radius 0.125
  circle A901 centre (-3, -1.5) radius 0.125
  circle A902 centre (-3, 0) radius 0.125
  circle A903 centre (-3, -0.5) radius 0.125
  circle A904 centre (-3, -1) radius 0.125
  circle A905 centre (-3, -9) radius 0.125
  circle A906 centre (-3, -8.5) radius 0.125
  circle A907 centre (-3, -8) radius 0.125
  circle A908 centre (-3, 3.5) radius 0.125
  circle A909 centre (-3, 4) radius 0.125
  circle A910 centre (-3, 4.5) radius 0.125
  circle A911 centre (-3, 7) radius 0.125
  circle A912 centre (-3, 7.5) radius 0.125
  circle A913 centre (-3, 8) radius 0.125
  circle A914 centre (-3, 8.5) radius 0.125
  circle A915 centre (-3, 9) radius 0.125
  circle A916 centre (-3, 0.5) radius 0.125
  circle A917 centre (-3, 1) radius 0.125
  circle A918 centre (-3, 1.5) radius 0.125
  circle A919 centre (-3, 2) radius 0.125
  circle A920 centre (-3, 2.5) radius 0.125
  circle A921 centre (-3, 3) radius 0.125
  circle A922 centre (-3, 5) radius 0.125
  circle A923 centre (-3, 5.5) radius 0.125
  circle A924 centre (-3, 6) radius 0.125
  circle A925 centre (-3, 6.5) radius 0.125
  line L8 (-3.5, -9) -> (-3.5, 0) construction
  circle A926 centre (-3.5, -5.5) radius 0.125
  circle A927 centre (-3.5, -5) radius 0.125
  circle A928 centre (-3.5, -3.5) radius 0.125
  circle A929 centre (-3.5, -4) radius 0.125
  circle A930 centre (-3.5, -4.5) radius 0.125
  circle A931 centre (-3.5, -7.5) radius 0.125
  circle A932 centre (-3.5, -7) radius 0.125
  circle A933 centre (-3.5, -6.5) radius 0.125
  circle A934 centre (-3.5, -6) radius 0.125
  circle A935 centre (-3.5, -3) radius 0.125
  circle A936 centre (-3.5, -2.5) radius 0.125
  circle A937 centre (-3.5, -2) radius 0.125
  circle A938 centre (-3.5, -1.5) radius 0.125
  circle A939 centre (-3.5, 0) radius 0.125
  circle A940 centre (-3.5, -0.5) radius 0.125
  circle A941 centre (-3.5, -1) radius 0.125
  circle A942 centre (-3.5, -9) radius 0.125
  circle A943 centre (-3.5, -8.5) radius 0.125
  circle A944 centre (-3.5, -8) radius 0.125
  circle A945 centre (-3.5, 3.5) radius 0.125
  circle A946 centre (-3.5, 4) radius 0.125
  circle A947 centre (-3.5, 4.5) radius 0.125
  circle A948 centre (-3.5, 7) radius 0.125
  circle A949 centre (-3.5, 7.5) radius 0.125
  circle A950 centre (-3.5, 8) radius 0.125
  circle A951 centre (-3.5, 8.5) radius 0.125
  circle A952 centre (-3.5, 9) radius 0.125
  circle A953 centre (-3.5, 0.5) radius 0.125
  circle A954 centre (-3.5, 1) radius 0.125
  circle A955 centre (-3.5, 1.5) radius 0.125
  circle A956 centre (-3.5, 2) radius 0.125
  circle A957 centre (-3.5, 2.5) radius 0.125
  circle A958 centre (-3.5, 3) radius 0.125
  circle A959 centre (-3.5, 5) radius 0.125
  circle A960 centre (-3.5, 5.5) radius 0.125
  circle A961 centre (-3.5, 6) radius 0.125
  circle A962 centre (-3.5, 6.5) radius 0.125
  line L9 (-4, -9) -> (-4, 0) construction
  circle A963 centre (-4, -5.5) radius 0.125
  circle A964 centre (-4, -5) radius 0.125
  circle A965 centre (-4, -3.5) radius 0.125
  circle A966 centre (-4, -4) radius 0.125
  circle A967 centre (-4, -4.5) radius 0.125
  circle A968 centre (-4, -7.5) radius 0.125
  circle A969 centre (-4, -7) radius 0.125
  circle A970 centre (-4, -6.5) radius 0.125
  circle A971 centre (-4, -6) radius 0.125
  circle A972 centre (-4, -3) radius 0.125
  circle A973 centre (-4, -2.5) radius 0.125
  circle A974 centre (-4, -2) radius 0.125
  circle A975 centre (-4, -1.5) radius 0.125
  circle A976 centre (-4, 0) radius 0.125
  circle A977 centre (-4, -0.5) radius 0.125
  circle A978 centre (-4, -1) radius 0.125
  circle A979 centre (-4, -9) radius 0.125
  circle A980 centre (-4, -8.5) radius 0.125
  circle A981 centre (-4, -8) radius 0.125
  circle A982 centre (-4, 3.5) radius 0.125
  circle A983 centre (-4, 4) radius 0.125
  circle A984 centre (-4, 4.5) radius 0.125
  circle A985 centre (-4, 7) radius 0.125
  circle A986 centre (-4, 7.5) radius 0.125
  circle A987 centre (-4, 8) radius 0.125
  circle A988 centre (-4, 8.5) radius 0.125
  circle A989 centre (-4, 9) radius 0.125
  circle A990 centre (-4, 0.5) radius 0.125
  circle A991 centre (-4, 1) radius 0.125
  circle A992 centre (-4, 1.5) radius 0.125
  circle A993 centre (-4, 2) radius 0.125
  circle A994 centre (-4, 2.5) radius 0.125
  circle A995 centre (-4, 3) radius 0.125
  circle A996 centre (-4, 5) radius 0.125
  circle A997 centre (-4, 5.5) radius 0.125
  circle A998 centre (-4, 6) radius 0.125
  circle A999 centre (-4, 6.5) radius 0.125
  line L10 (-4.5, -9) -> (-4.5, 0) construction
  circle A1000 centre (-4.5, -5.5) radius 0.125
  circle A1001 centre (-4.5, -5) radius 0.125
  circle A1002 centre (-4.5, -3.5) radius 0.125
  circle A1003 centre (-4.5, -4) radius 0.125
  circle A1004 centre (-4.5, -4.5) radius 0.125
  circle A1005 centre (-4.5, -7.5) radius 0.125
  circle A1006 centre (-4.5, -7) radius 0.125
  circle A1007 centre (-4.5, -6.5) radius 0.125
  circle A1008 centre (-4.5, -6) radius 0.125
  circle A1009 centre (-4.5, -3) radius 0.125
  circle A1010 centre (-4.5, -2.5) radius 0.125
  circle A1011 centre (-4.5, -2) radius 0.125
  circle A1012 centre (-4.5, -1.5) radius 0.125
  circle A1013 centre (-4.5, 0) radius 0.125
  circle A1014 centre (-4.5, -0.5) radius 0.125
  circle A1015 centre (-4.5, -1) radius 0.125
  circle A1016 centre (-4.5, -9) radius 0.125
  circle A1017 centre (-4.5, -8.5) radius 0.125
  circle A1018 centre (-4.5, -8) radius 0.125
  circle A1019 centre (-4.5, 3.5) radius 0.125
  circle A1020 centre (-4.5, 4) radius 0.125
  circle A1021 centre (-4.5, 4.5) radius 0.125
  circle A1022 centre (-4.5, 7) radius 0.125
  circle A1023 centre (-4.5, 7.5) radius 0.125
  circle A1024 centre (-4.5, 8) radius 0.125
  circle A1025 centre (-4.5, 8.5) radius 0.125
  circle A1026 centre (-4.5, 9) radius 0.125
  circle A1027 centre (-4.5, 0.5) radius 0.125
  circle A1028 centre (-4.5, 1) radius 0.125
  circle A1029 centre (-4.5, 1.5) radius 0.125
  circle A1030 centre (-4.5, 2) radius 0.125
  circle A1031 centre (-4.5, 2.5) radius 0.125
  circle A1032 centre (-4.5, 3) radius 0.125
  circle A1033 centre (-4.5, 5) radius 0.125
  circle A1034 centre (-4.5, 5.5) radius 0.125
  circle A1035 centre (-4.5, 6) radius 0.125
  circle A1036 centre (-4.5, 6.5) radius 0.125
  line L11 (-5, -9) -> (-5, 0) construction
  circle A1037 centre (-5, -5.5) radius 0.125
  circle A1038 centre (-5, -5) radius 0.125
  circle A1039 centre (-5, -3.5) radius 0.125
  circle A1040 centre (-5, -4) radius 0.125
  circle A1041 centre (-5, -4.5) radius 0.125
  circle A1042 centre (-5, -7.5) radius 0.125
  circle A1043 centre (-5, -7) radius 0.125
  circle A1044 centre (-5, -6.5) radius 0.125
  circle A1045 centre (-5, -6) radius 0.125
  circle A1046 centre (-5, -3) radius 0.125
  circle A1047 centre (-5, -2.5) radius 0.125
  circle A1048 centre (-5, -2) radius 0.125
  circle A1049 centre (-5, -1.5) radius 0.125
  circle A1050 centre (-5, 0) radius 0.125
  circle A1051 centre (-5, -0.5) radius 0.125
  circle A1052 centre (-5, -1) radius 0.125
  circle A1053 centre (-5, -9) radius 0.125
  circle A1054 centre (-5, -8.5) radius 0.125
  circle A1055 centre (-5, -8) radius 0.125
  circle A1056 centre (-5, 3.5) radius 0.125
  circle A1057 centre (-5, 4) radius 0.125
  circle A1058 centre (-5, 4.5) radius 0.125
  circle A1059 centre (-5, 7) radius 0.125
  circle A1060 centre (-5, 7.5) radius 0.125
  circle A1061 centre (-5, 8) radius 0.125
  circle A1062 centre (-5, 8.5) radius 0.125
  circle A1063 centre (-5, 9) radius 0.125
  circle A1064 centre (-5, 0.5) radius 0.125
  circle A1065 centre (-5, 1) radius 0.125
  circle A1066 centre (-5, 1.5) radius 0.125
  circle A1067 centre (-5, 2) radius 0.125
  circle A1068 centre (-5, 2.5) radius 0.125
  circle A1069 centre (-5, 3) radius 0.125
  circle A1070 centre (-5, 5) radius 0.125
  circle A1071 centre (-5, 5.5) radius 0.125
  circle A1072 centre (-5, 6) radius 0.125
  circle A1073 centre (-5, 6.5) radius 0.125
  line L12 (-5.5, -9) -> (-5.5, 0) construction
  circle A1074 centre (-5.5, -5.5) radius 0.125
  circle A1075 centre (-5.5, -5) radius 0.125
  circle A1076 centre (-5.5, -3.5) radius 0.125
  circle A1077 centre (-5.5, -4) radius 0.125
  circle A1078 centre (-5.5, -4.5) radius 0.125
  circle A1079 centre (-5.5, -7.5) radius 0.125
  circle A1080 centre (-5.5, -7) radius 0.125
  circle A1081 centre (-5.5, -6.5) radius 0.125
  circle A1082 centre (-5.5, -6) radius 0.125
  circle A1083 centre (-5.5, -3) radius 0.125
  circle A1084 centre (-5.5, -2.5) radius 0.125
  circle A1085 centre (-5.5, -2) radius 0.125
  circle A1086 centre (-5.5, -1.5) radius 0.125
  circle A1087 centre (-5.5, 0) radius 0.125
  circle A1088 centre (-5.5, -0.5) radius 0.125
  circle A1089 centre (-5.5, -1) radius 0.125
  circle A1090 centre (-5.5, -9) radius 0.125
  circle A1091 centre (-5.5, -8.5) radius 0.125
  circle A1092 centre (-5.5, -8) radius 0.125
  circle A1093 centre (-5.5, 3.5) radius 0.125
  circle A1094 centre (-5.5, 4) radius 0.125
  circle A1095 centre (-5.5, 4.5) radius 0.125
  circle A1096 centre (-5.5, 7) radius 0.125
  circle A1097 centre (-5.5, 7.5) radius 0.125
  circle A1098 centre (-5.5, 8) radius 0.125
  circle A1099 centre (-5.5, 8.5) radius 0.125
  circle A1100 centre (-5.5, 9) radius 0.125